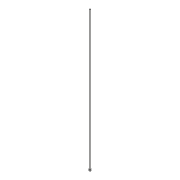
# Autodesk Inventor part: 6m_GENERIC_FLAT
Saved by Autodesk Inventor 2017 (Build 210142000, 142)
## iProperties
Created: 2017-03-09
Part Number: 6m_GENERIC_FLAT
Material: Generic
Document SubType Name: Modeling
Designer: krosie
Density: 1 g/cm^3
Appearance: Default
Author: krosie
Autodesk Inventor part; units mm, degrees
ref_plane "YZ Plane" through (0, 0, 0) normal (1, 0, 0) x (0, 1, 0)
ref_plane "XZ Plane" through (0, 0, 0) normal (0, 1, 0) x (-1, 0, 0)
ref_plane "XY Plane" through (0, 0, 0) normal (0, 0, 1) x (1, 0, 0)
sketch "Sketch1" plane through (0, 0, 0) normal (0, 0, 1) x (1, 0, 0)
  circle A0 centre (0, 0) radius 31.5
  circle A1 centre (0, 0) radius 27.9
  dimension "d0" = 63
  dimension "d1" = 3.6
  constraints: 2 centre point, 2 coincident
  measures "d0" diameter of A0
  measures "d1" radial gap between concentric circles of A0 A1
extrude "Extrusion1" add sketch "Sketch1" along normal blind 6000
sketch "Sketch2" plane through (0, 0, 0) normal (1, 0, 0) x (0, 1, 0)
  line L0 (27.9, 0) -> (38.7, 0)
  line L1 (38.7, 0) -> (38.7, -38.7)
  line L2 (48.7, -46.2) -> (48.7, -46.2)
  line L3 (38.7, -53.7) -> (38.7, -68.7)
  arc A0 (48.7, -46.2) -> (41.2, -38.7) centre (41.2, -46.2) ccw
  arc A1 (41.2, -53.7) -> (48.7, -46.2) centre (41.2, -46.2) ccw
  line L4 (41.2, -38.7) -> (38.7, -38.7)
  line L5 (41.2, -53.7) -> (38.7, -53.7)
  line L6 (31.5, 6000) -> (-31.5, 6000) projected
  line L7 (-31.5, 0) -> (31.5, 0) projected
  line L8 (27.9, 0) -> (27.9, -5.2)
  line L9 (0, -1282.44) -> (0, 7213.74) projected
  line L10 (31.5, -68.7) -> (31.5, -5.2)
  line L11 (31.5, -5.2) -> (27.9, -5.2)
  line L12 (31.5, -68.7) -> (38.7, -68.7)
  point P0 (0, 0)
  point P1 (48.7, -53.7)
  point P2 (48.7, -38.7)
  dimension "d4" = 38.7
  dimension "d6" = 15
  dimension "d7" = 10
  dimension "d8" = 15
  dimension "d9" = 7.5
  dimension "d12" = 3.6
  dimension "d13" = 63.5
  constraints: 20 end point, 4 point on circle, 3 point on line, 2 centre point, 2 perpendicular, 2 tangent, 1 concentric, 1 horizontal, 1 parallel
  measures "d4" distance of L0.end L1.end
  measures "d6" distance of point (48.7, -38.7) point (48.7, -53.7)
  measures "d7" distance between parallel lines of L1 L2
  measures "d8" distance of L3.start L3.end
  measures "d9" radius of A0
  measures "d12" distance of L8.end L10.end
  measures "d13" distance of L10.end L10.start
revolve "Revolution1" add sketch "Sketch2" angle 360 about axis through (0, 0, -10) along (0, 0, 1)
fillet "Fillet4" radius 5 2 edges at (0, -38.7, -53.7) (0, -38.7, -38.7)
fillet "Fillet5" radius 5 2 edges at (-31.5, 0, 0) (0, -38.7, 0)
body "Solid1"
